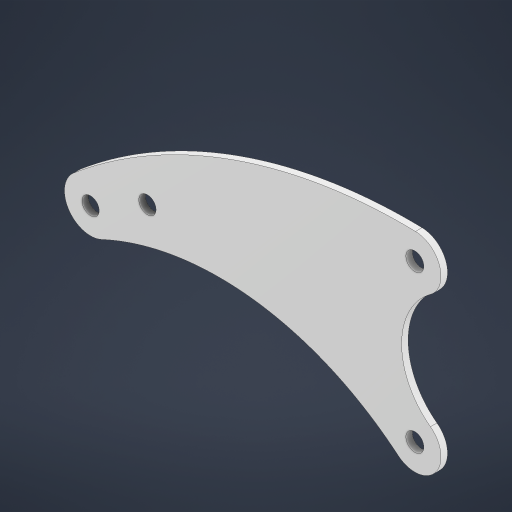
# Autodesk Inventor part: triball_jig
Saved by Autodesk Inventor 2024 (Build 280153000, 153)
## iProperties
Created: 2023-11-21
Part Number: triball_jig
Material: Acetal Resin, White
Document SubType Name: Sheet Metal
Designer: avere
Density: 1.425 g/cm^3
Appearance: Smooth - White
Flat Pattern Width: 5.07905 cm
Flat Pattern Length: 9.1839 cm
Flat Pattern Area: 46.6455 cm^2
Sheet Metal Rule: Default_mm
Sheet Metal Width: 2.000 in
Sheet Metal Length: 3.616 in
Sheet Metal Area: 7.230 in^2
Author: avere
Autodesk Inventor part; units mm, degrees
ref_plane "YZ Plane" through (0, 0, 0) normal (1, 0, 0) x (0, 1, 0)
ref_plane "XZ Plane" through (0, 0, 0) normal (0, 1, 0) x (-1, 0, 0)
ref_plane "XY Plane" through (0, 0, 0) normal (0, 0, 1) x (1, 0, 0)
sketch "Block1" plane through (0, 0, 0) normal (0, 0, 1) x (1, 0, 0)
  circle A0 centre (47.0944, 34.7657) radius 2.1844
  circle A1 centre (-31.8333, 45.0945) radius 2.0955
  arc A2 (-35.9193, 49.9553) -> (-29.157, 39.3361) centre (-31.8333, 45.0945) ccw
  arc A3 (43.0264, 29.8899) -> (53.4444, 34.7657) centre (47.0944, 34.7657) ccw
  arc A4 (43.0264, 29.8899) -> (-29.157, 39.3361) centre (-0.5124, -22.2949) ccw
  circle A5 centre (47.0944, 72.8657) radius 2.1844
  arc A6 (53.4444, 72.8657) -> (47.2364, 79.2141) centre (47.0944, 72.8657) ccw
  arc A7 (47.2364, 79.2141) -> (-35.9193, 49.9553) centre (44.4441, -45.6465) ccw
  circle A8 centre (-17.9931, 52.2282) radius 2.0955
  point P0 (37.587, 35.3505)
  dimension "d2" = 12.7
  dimension "d3" = 12.7
  dimension "d4" = 12.7
  dimension "d9" = 4.191
  measures "d2" diameter of A2
  measures "d3" diameter of A3
  measures "d4" diameter of A6
  measures "d9" diameter of A8
sketch "Sketch1" plane through (0, 0, 0) normal (0, 0, 1) x (1, 0, 0)
  arc A0 (3.787, 33.0028) -> (0.142, 44.4484) centre (0, 38.1) ccw
  arc A1 (-4.068, -4.8758) -> (3.787, 5.0972) centre (0, 0) ccw
  arc A2 (3.787, 33.0028) -> (3.787, 5.0972) centre (14.1532, 19.05) ccw
  circle A3 centre (0, 0) radius 2.1844
  circle A4 centre (-78.9278, 10.3288) radius 2.0955
  arc A5 (-83.0138, 15.1896) -> (-76.2514, 4.5703) centre (-78.9278, 10.3288) ccw
  arc A6 (-4.068, -4.8758) -> (6.35, 0) centre (0, 0) ccw
  arc A7 (-4.068, -4.8758) -> (-76.2514, 4.5703) centre (-47.6069, -57.0606) ccw
  circle A8 centre (0, 38.1) radius 2.1844
  arc A9 (6.35, 38.1) -> (0.142, 44.4484) centre (0, 38.1) ccw
  arc A10 (0.142, 44.4484) -> (-83.0138, 15.1896) centre (-2.6504, -80.4122) ccw
  circle A11 centre (-65.0875, 17.4625) radius 2.0955
  point P0 (6.35, 0)
  point P1 (6.35, 38.1)
  constraints: 6 point on circle, 3 centre point, 2 tangent, 6 other
extrude "Extrusion1" add sketch "Sketch1" along normal blind 1.5875
equation "\"BendRadius\" = Thickness"
equation "\"BendReliefWidth\" = Thickness"
equation "\"BendReliefDepth\" = 0.5 * Thickness"
equation "\"CornerReliefSize\" = 4 * Thickness"
equation "\"MinimumRemnant\" = 2 * Thickness"
equation "\"TransitionRadius\" = BendRadius"
equation "\"JacobiRadiusSize\" = BendRadius"
equation "\"GapSize\" = Thickness"
equation "\"Thickness\" = 1.5875"
body "Solid1"
